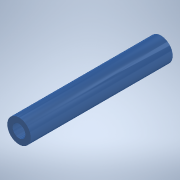
# Autodesk Inventor part: Spacer3_8x1.27
Saved by Autodesk Inventor 2020 (Build 240168000, 168)
## iProperties
Created: 2020-01-19
Part Number: Spacer3_8x1.27
Material: Generic
Document SubType Name: Modeling
Designer: srini
Density: 1 g/cm^3
Appearance: Flaked Satin - Blue
Author: srini
Autodesk Inventor part; units mm, degrees
ref_plane "YZ Plane" through (0, 0, 0) normal (1, 0, 0) x (0, 1, 0)
ref_plane "XZ Plane" through (0, 0, 0) normal (0, 1, 0) x (-1, 0, 0)
ref_plane "XY Plane" through (0, 0, 0) normal (0, 0, 1) x (1, 0, 0)
sketch "Sketch1" plane through (0, 0, 0) normal (0, 0, 1) x (1, 0, 0)
  circle A0 centre (0, 0) radius 2.5781
  circle A1 centre (0, 0) radius 4.7625
  dimension "d0" = 5.1562
  dimension "d1" = 9.525
  constraints: 2 centre point, 2 coincident
  measures "d0" diameter of A0
  measures "d1" diameter of A1
extrude "Extrusion1" add sketch "Sketch1" along normal blind 57.658
body "Solid1"
